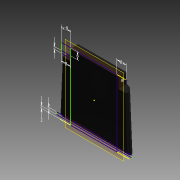
# Autodesk Inventor part: astra_clip1
Saved by Autodesk Inventor 2015 (Build 190159000, 159)
## iProperties
Created: 2016-02-10
Part Number: astra_clip1
Material: Generic
Document SubType Name: Modeling
Designer: John
Density: 1 g/cm^3
Appearance: Default
Author: John
Autodesk Inventor part; units mm, degrees
ref_plane "YZ Plane" through (0, 0, 0) normal (1, 0, 0) x (0, 1, 0)
ref_plane "XZ Plane" through (0, 0, 0) normal (0, 1, 0) x (-1, 0, 0)
ref_plane "XY Plane" through (0, 0, 0) normal (0, 0, 1) x (1, 0, 0)
sketch "Sketch3" plane through (0, 0, 0) normal (0, 1, 0) x (-1, 0, 0)
  line L0 (30, 29) -> (-30, 29)
  line L1 (-30, 29) -> (-30, -29)
  line L2 (-30, -29) -> (30, -29)
  line L3 (30, -29) -> (30, 29)
  line L4 (30, 29) -> (-30, -29) construction
  line L5 (-30, 29) -> (30, -29) construction
  line L6 (-27.5, 29) -> (27.5, 29)
  line L7 (-27.5, 29) -> (-30, -29)
  line L8 (27.5, 29) -> (30, -29)
  point P0 (0, 0)
  dimension "d7" = 60
  dimension "d8" = 58
  dimension "d9" = 2.5
  dimension "d10" = 2.5
  constraints: 19 end point, 2 midpoint, 2 parallel, 2 point on line, 1 horizontal, 1 perpendicular
  measures "d7" distance of L1.end L2.end
  measures "d8" distance of L1.end L0.end
  measures "d9" distance of L6.end L0.start
  measures "d10" distance of L0.end L6.start
extrude "Extrusion2" add sketch "Sketch3" along normal blind 14 contours L8 L2 L7 L0
fillet "Fillet1" radius 7 4 edges at (-28.75, 14, 0) (-28.75, 0, 0) (28.75, 14, 0) (28.75, 0, 0)
ref_plane "Work Plane2" through (0, 7, 0) normal (0, -1, 0) x (1, 0, 0)
sketch "Sketch13" plane through (0, 7, 0) normal (0, -1, 0) x (1, 0, 0)
  line L0 (-22.9935, -29) -> (-30, -29) projected
  line L1 (30, -29) -> (22.9935, -29) projected
  line L2 (-27.5, 29) -> (-20.4935, 29) projected
  line L3 (20.4935, 29) -> (27.5, 29) projected
  line L4 (-28.4935, 23) -> (-20.4935, 23)
  line L5 (-20.4935, 23) -> (-20.4935, 29)
  line L6 (-20.4935, 29) -> (-28.4935, 29)
  line L7 (-28.4935, 29) -> (-28.4935, 23)
  line L8 (-20.4935, 29) -> (20.4935, 29) projected
  line L9 (-20.4935, 23) -> (-28.4935, 23)
  line L10 (-28.4935, 23) -> (-28.4935, 21)
  line L11 (-28.4935, 21) -> (-20.4935, 21)
  line L12 (-20.4935, 21) -> (-20.4935, 23)
  line L13 (22.9935, -29) -> (-22.9935, -29) projected
  line L14 (-20.4935, 29) -> (19.5, 29)
  line L15 (19.5, 29) -> (19.5, -29)
  line L16 (19.5, -29) -> (-20.4935, -29)
  line L17 (-20.4935, -29) -> (-20.4935, 29)
  line L18 (-20.4935, 29) -> (19.5, 29)
  line L19 (19.5, 29) -> (19.5, -29)
  line L20 (19.5, -29) -> (-20.4935, -29)
  line L21 (-20.4935, -29) -> (-20.4935, 29)
  line L22 (-32.9403, -27) -> (32.541, -27)
  line L23 (32.541, -27) -> (32.541, -25)
  line L24 (32.541, -25) -> (-32.9403, -25)
  line L25 (-32.9403, -25) -> (-32.9403, -27)
  point P0 (0, 0)
  dimension "d57" = 6
  dimension "d58" = 8
  dimension "d59" = 8
  dimension "d60" = 2
  dimension "d61" = 8
  dimension "d62" = 2
  dimension "d63" = 2
  constraints: 40 end point, 10 parallel, 5 horizontal, 5 perpendicular, 1 coincident, 1 collinear, 1 point on line
  measures "d57" distance of L5.end L4.end
  measures "d58" distance of L5.end L6.end
  measures "d59" distance of L11.end L10.end
  measures "d60" distance of L10.end L9.end
  measures "d61" distance from line of L15 point (27.5, 29)
  measures "d62" distance of L24.end L22.start
  measures "d63" distance between parallel lines of L16 L22
sketch "Sketch14" plane through (22.9935, 0, -29) normal (0, 0, -1) x (-1, 0, 0)
  ellipse E0 centre (0, 7) end of major axis (-7.0065, 7) minor radius 7 (0, 14) -> (0, 0) ccw projected
  line L0 (0, 0) -> (45.987, 0) projected
  ellipse E1 centre (45.987, 7) end of major axis (52.9935, 7) minor radius 7 (45.987, 0) -> (45.987, 14) ccw projected
  line L1 (0, 14) -> (45.987, 14) projected
  ellipse E2 centre (0, 7) end of major axis (-7.0065, 7) minor radius 7 (0, 14) -> (0, 0) ccw projected
  line L2 (-7.0053, 6.868) -> (52.9935, 6.9757)
  ellipse E3 centre (45.987, 7) end of major axis (52.9935, 7) minor radius 7 (45.987, 0) -> (45.987, 14) ccw projected
  point P0 (22.9935, 0)
  constraints: 2 end point, 8 other
extrude "Extrusion11" cut sketch "Sketch14" against normal up to next contours L2 E1 L0 E0
fillet "Fillet6" radius 5 1 edges at (-0.0006, 6.9219, -29)
fillet "Fillet7" radius 1 7 edges at (-29.7558, 8.6115, -27.6994) (-25.6603, 13.4732, -29) (0, 14, -29) (25.7255, 13.446, -29) (29.724, 8.7786, -27.931) (28.641, 6.8704, 2.4999) (-28.6422, 6.9733, 2.5)
sketch "Sketch15" plane through (0, 14, 0) normal (0, 1, 0) x (1, 0, 0)
  line L0 (22.9504, 28) -> (27.0348, 27.9749) projected
  line L1 (22.9504, 28) -> (20.4935, -29) projected
  line L2 (20.4935, -29) -> (27.4252, -29) projected
  line L3 (-27.408, -29) -> (-20.4935, -29) projected
  line L4 (-20.4935, -29) -> (-22.9504, 28) projected
  line L5 (-26.8762, 27.9759) -> (-22.9504, 28) projected
  line L6 (-22.9504, 28) -> (22.9504, 28) projected
  line L7 (-20.4935, -29) -> (-22.9504, 28) projected
  line L8 (-20.4935, -29) -> (20.4935, -29) projected
  line L9 (22.9504, 28) -> (20.4935, -29) projected
  line L10 (-20.4935, -29) -> (20.4935, -29) projected
  line L11 (0, -29) -> (21, -29)
  line L12 (21, -29) -> (31, -29)
  line L13 (31, -29) -> (31, -19)
  line L14 (31, -19) -> (21, -19)
  line L15 (21, -19) -> (21, -29)
  line L16 (0, -29) -> (0, -33.3863) construction
  line L17 (-20.4935, -29) -> (-27.4252, -29)
  line L18 (-21, -29) -> (-31, -29)
  line L19 (-31, -29) -> (-31, -19)
  line L20 (-31, -19) -> (-21, -19)
  line L21 (-21, -19) -> (-21, -29)
  point P0 (0, 0)
  dimension "d69" = 21
  dimension "d70" = 10
  dimension "d71" = 10
  constraints: 22 end point, 7 symmetric about line, 2 parallel, 2 point on line, 1 horizontal, 1 midpoint, 1 perpendicular, 1 vertical, 4 other
  measures "d69" distance of L11.start L11.end
  measures "d70" distance of L14.end L13.end
  measures "d71" distance of L13.end L12.end
extrude "Extrusion12" cut sketch "Sketch15" against normal up to surface contours L15 L14 L13 L12 L2 | L17 L18 L19 L20 L21 L3 surface through (29.9988, 6.868, -29) normal (0.0017951, 0.9999984, 0)
sketch "Sketch16" plane through (-21, 6.9596, 19) normal (-1, 0, 0) x (0, 0, 1)
  ellipse E0 centre (-1.7508, 0.0404) end of major axis (160.8, 0.0404) minor radius 7 (10, 7.0221) -> (0, 7.04) ccw projected
  line L0 (0, 7.04) -> (0, 0) projected
  line L1 (10, 0) -> (0, 0) projected
  line L2 (10, 7.0221) -> (10, 0) projected
  circle A0 centre (5, 3.5111) radius 1.5
  point P0 (-19, -6.9596)
  dimension "d74" = 3
  constraints: 1 centre point, 1 other
  measures "d74" diameter of A0
extrude "Extrusion13" cut sketch "Sketch16" against normal up to next contours A0
sketch "Sketch17" plane through (-20.4935, 14, 29) normal (0, 0, 1) x (1, 0, 0)
  line L0 (-0.5065, -0.0183) -> (-0.5065, -7.0404) projected
  line L1 (-0.5065, -7.0404) -> (41.4935, -7.1158) projected
  line L2 (41.4935, -7.1158) -> (41.4935, -0.0183) projected
  ellipse E0 centre (40.987, -7) end of major axis (47.9935, -7) minor radius 7 (41.4935, -0.0183) -> (40.987, 0) ccw projected
  line L3 (0, 0) -> (40.987, 0) projected
  ellipse E1 centre (0, -7) end of major axis (-7.0065, -7) minor radius 7 (0, 0) -> (-0.5065, -0.0183) ccw projected
  line L4 (41.9935, -7.5671) -> (-1.0065, -7.5671)
  line L5 (-1.0065, -7.5671) -> (-1.0065, 0.4329)
  line L6 (-1.0065, 0.4329) -> (41.9935, 0.4329)
  line L7 (41.9935, 0.4329) -> (41.9935, -7.5671)
  line L8 (41.9935, -7.5671) -> (-1.0065, 0.4329) construction
  line L9 (-1.0065, -7.5671) -> (41.9935, 0.4329) construction
  point P0 (20.4935, -14)
  point P1 (20.4935, -3.5671)
  dimension "d77" = 43
  dimension "d78" = 8
  constraints: 12 end point, 2 midpoint, 2 parallel, 1 horizontal, 1 perpendicular, 2 other
  measures "d77" distance of L5.end L6.end
  measures "d78" distance of L4.end L5.end
extrude "Extrusion14" cut sketch "Sketch17" against normal blind 1 contours E1 L3 E0 L2 L1 L0 | L4 L5 L6 L7
sketch "Sketch18" plane through (0, 14, 0) normal (0, 1, 0) x (1, 0, 0)
  circle A0 centre (0, 11) radius 2.5
  line L0 (28.7182, 24) -> (-28.7058, 24) projected
  line L1 (-22.9504, 29) -> (-26.3163, 29) projected
  line L2 (22.9504, 29) -> (-22.9504, 29) projected
  line L3 (26.4523, 29) -> (22.9504, 29) projected
  line L4 (-26.3163, 29) -> (26.4523, 29) projected
  point P0 (0, 0)
  dimension "d81" = 5
  dimension "d82" = 18
  constraints: 1 centre point, 1 coincident
  measures "d81" diameter of A0
  measures "d82" distance from line of A0.centre L4
extrude "Extrusion15" cut sketch "Sketch18" against normal blind 5
thread "Thread1" size "M5x0.8" class "6H" standard "ANSI Metric M Profile" full length
equation "\"d10\" = d9"
equation "\"d58\" = d61"
body "Solid2"
